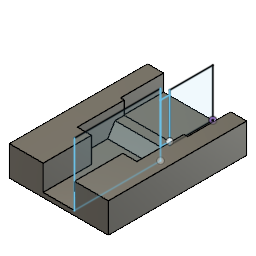
Universal Power v1 (Autodesk Fusion 360 design; units mm, degrees)
Autodesk Fusion 360 part; units mm, degrees
sketch "Sketch1" plane through (0, 0, 0) normal (1, 0, 0) x (0, 0, -1)
  line L0 (0, 0) -> (-18.75, 0)
  line L1 (-18.75, 0) -> (-18.75, 20.75)
  line L2 (-18.75, 20.75) -> (0, 20.75)
  line L3 (0, 20.75) -> (0, 0)
  line L4 (-18.75, 20.75) -> (-18.75, 19)
  line L5 (-18.75, 0) -> (-18.75, 1.4)
  line L6 (-18.75, 19) -> (-22.75, 19)
  line L7 (-22.75, 19) -> (-22.75, 1.4)
  line L8 (-22.75, 1.4) -> (-18.75, 1.4)
  line L9 (-18.75, 1.4) -> (-18.75, 19)
  line L10 (-22.75, 19) -> (-22.75, 23.35)
  line L11 (-22.75, 1.4) -> (-22.75, -3.85)
  line L12 (-22.75, 23.35) -> (-60.15, 23.35)
  line L13 (-60.15, 23.35) -> (-60.15, -3.85)
  line L14 (-60.15, -3.85) -> (-22.75, -3.85)
  line L15 (-22.75, -3.85) -> (-22.75, 23.35)
  dimension "d1" = 18.75
  dimension "d2" = 20.75
  dimension "d4" = 1.75
  dimension "d6" = 4
  dimension "d7" = 4.35
  dimension "d9" = 37.4
  constraint horizontal L0
  constraint vertical L1
  constraint horizontal L2
  constraint vertical L3
  constraint coincident L0.start L3.end
  constraint horizontal L6
  constraint vertical L7
  constraint horizontal L8
  constraint vertical L9
  constraint horizontal L12
  constraint vertical L13
  constraint horizontal L14
  constraint vertical L15
  measures "d1" distance of L0.start L0.end
  measures "d2" distance of L0.start L2.end
  measures "d4" distance of L1.end L4.end
  measures "d6" distance of L4.end L6.end
  measures "d7" distance of L6.end L10.end
  measures "d9" distance of L10.end L12.end
sketch "Sketch3" plane through (0, 0, 0) normal (1, 0, 0) x (0, 0, -1)
  line L0 (-60.15, -3.85) -> (-60.15, 7.15)
  line L1 (-60.15, 7.15) -> (-39.15, 7.15)
  line L2 (-60.15, -3.85) -> (-22.75, -3.85)
  line L3 (-39.15, 7.15) -> (-39.15, -3.85)
  point P0 (-60.15, -3.85)
  dimension "d10" = 11
  dimension "d11" = 21
  constraint coincident P0 L0.start
  constraint coincident L2 L3.end
  constraint perpendicular L1 L3
  measures "d10" distance of P0 L0.end
  measures "d11" distance of L0.end L1.end
extrude "Extrude1" add sketch "Sketch3" along normal blind 6.15 makes body 1
sketch "Sketch4" plane through (6.15, 0, 0) normal (1, 0, 0) x (0, 0, -1)
  line L0 (-60.15, -3.85) -> (-39.15, -3.85)
  line L1 (-39.15, -3.85) -> (-39.15, 7.15)
  line L2 (-39.15, 7.15) -> (-60.15, 7.15)
  line L3 (-60.15, 7.15) -> (-60.15, -3.85)
  line L4 (-60.15, -3.85) -> (-18.75, -3.85)
  line L5 (-18.75, -3.85) -> (-18.75, 7.15)
  line L6 (-18.75, 7.15) -> (-60.15, 7.15)
  line L7 (-60.15, 7.15) -> (-60.15, -3.85)
  line L8 (-18.75, 1.4) -> (-18.75, 19)
  constraint horizontal L4
  constraint vertical L5
  constraint horizontal L6
  constraint vertical L7
  constraint coincident L5.end L8
  constraint coincident L0.start L3.end
extrude "Extrude2" add sketch "Sketch4" along normal blind 1.6 bodies 1
sketch "Sketch5" plane through (7.75, 0, 0) normal (1, 0, 0) x (0, 0, -1)
  line L0 (-18.75, -3.85) -> (-18.75, 7.15)
  line L1 (-18.75, 7.15) -> (-60.15, 7.15)
  line L2 (-60.15, 7.15) -> (-60.15, -3.85)
  line L3 (-60.15, -3.85) -> (-18.75, -3.85)
  line L4 (-60.15, -3.85) -> (0, -3.85)
  line L5 (0, -3.85) -> (0, 7.15)
  line L6 (0, 7.15) -> (-60.15, 7.15)
  line L7 (-60.15, 7.15) -> (-60.15, -3.85)
  line L8 (0, 20.75) -> (0, 0)
  constraint horizontal L4
  constraint vertical L5
  constraint horizontal L6
  constraint vertical L7
  constraint coincident L5.end L8
  constraint coincident L2.end L3.start
extrude "Extrude3" add sketch "Sketch5" along normal blind 7 bodies 1
sketch "Sketch6" plane through (0, 0, 60.15) normal (0, 0, 1) x (1, 0, 0)
  line L0 (0, 7.15) -> (0, -3.85)
  line L1 (0, -3.85) -> (14.75, -3.85)
  line L2 (14.75, -3.85) -> (14.75, 7.15)
  line L3 (14.75, 7.15) -> (0, 7.15)
  line L4 (0, -3.85) -> (-13.6, -3.85)
  dimension "d18" = 13.6
  constraint coincident L0.end L1.start
  measures "d18" distance of L0.end L4.end
extrude "Extrude4" add sketch "Sketch3" along normal blind -14 and the other way blind 13.6 separate body makes body 2
extrude "Extrude5" add 1 faces at (-14, -0.1833, 46.15) along direction (-1, 0, 0) blind 6.15 on bodies 2 bodies 2
extrude "Extrude6" cut 1 faces at (-20.15, -0.1833, 46.15) along direction (1, 0, 0) blind 0.4 on bodies 2 bodies 2
sketch "Sketch7" plane through (-19.75, 0, 0) normal (-1, 0, 0) x (0, 0, 1)
  line L0 (39.15, -3.85) -> (60.15, -3.85)
  line L1 (60.15, -3.85) -> (60.15, 7.15)
  line L2 (60.15, 7.15) -> (39.15, 7.15)
  line L3 (39.15, 7.15) -> (39.15, -3.85)
  line L4 (60.15, 7.15) -> (18.75, 7.15)
  line L5 (18.75, 7.15) -> (18.75, -3.85)
  line L6 (18.75, -3.85) -> (60.15, -3.85)
  line L7 (60.15, -3.85) -> (60.15, 7.15)
  point P0 (18.75, -3.85)
  constraint horizontal L4
  constraint vertical L5
  constraint horizontal L6
  constraint vertical L7
  constraint coincident P0 L5.end
  constraint coincident L1.end L2.start
extrude "Extrude7" add sketch "Sketch7" along normal blind 1.6 bodies 2
sketch "Sketch8" plane through (-21.35, 0, 0) normal (-1, 0, 0) x (0, 0, 1)
  line L0 (60.15, -3.85) -> (60.15, 7.15)
  line L1 (60.15, 7.15) -> (18.75, 7.15)
  line L2 (18.75, 7.15) -> (18.75, -3.85)
  line L3 (18.75, -3.85) -> (60.15, -3.85)
  line L4 (60.15, 7.15) -> (0, 7.15)
  line L5 (0, 7.15) -> (0, -3.85)
  line L6 (0, -3.85) -> (60.15, -3.85)
  line L7 (60.15, -3.85) -> (60.15, 7.15)
  point P0 (0, -3.85)
  constraint horizontal L4
  constraint vertical L5
  constraint horizontal L6
  constraint vertical L7
  constraint coincident P0 L5.end
  constraint coincident L0.end L1.start
extrude "Extrude8" add sketch "Sketch8" along normal blind 7 bodies 2
sketch "Sketch9" plane through (0, 0, 0) normal (1, 0, 0) x (0, 0, -1)
  line L0 (-60.15, -3.85) -> (-25.95, -3.85)
  line L1 (-25.95, -3.85) -> (-22.75, 1.4)
  line L2 (-22.75, 1.4) -> (-18.75, 1.4)
  line L3 (-18.75, 1.4) -> (-18.75, 0)
  line L4 (-18.75, 0) -> (0, 0)
  line L5 (-25.95, -3.85) -> (0, -3.85)
  line L6 (0, -3.85) -> (0, 0)
  point P0 (-60.15, -3.85)
  point P1 (-22.75, 1.4)
  point P2 (-18.75, 1.4)
  point P3 (-18.75, 0)
  dimension "d31" = 34.2
  constraint coincident P0 L0.start
  constraint coincident P1 L1.end
  constraint coincident P2 L2.end
  constraint parallel L0 L2
  constraint coincident P3 L3.end
  constraint coincident L4.end L6.end
  constraint parallel L0 L5
  constraint perpendicular L4 L6
  measures "d31" distance of P0 L0.end
extrude "Extrude9" add sketch "Sketch9" along normal blind 8 and the other way blind 24 bodies 1 2
sketch "Sketch10" plane through (0, -3.85, 0) normal (0, -1, 0) x (1, 0, 0)
  line L0 (-19.75, 25.95) -> (-19.75, 39.15)
  line L1 (-19.75, 39.15) -> (-13.6, 39.15)
  line L2 (-13.6, 39.15) -> (-13.6, 60.15)
  line L3 (-13.6, 60.15) -> (-28.35, 60.15)
  line L4 (-28.35, 60.15) -> (-28.35, 0)
  line L5 (-28.35, 0) -> (14.75, 0)
  line L6 (14.75, 0) -> (14.75, 60.15)
  line L7 (14.75, 60.15) -> (0, 60.15)
  line L8 (0, 60.15) -> (0, 39.15)
  line L9 (0, 39.15) -> (6.15, 39.15)
  line L10 (6.15, 39.15) -> (6.15, 25.95)
  line L11 (6.15, 25.95) -> (-19.75, 25.95)
  line L12 (-28.35, 60.15) -> (14.75, 60.15)
  line L13 (14.75, 60.15) -> (14.75, 0)
  line L14 (14.75, 0) -> (-28.35, 0)
  line L15 (-28.35, 0) -> (-28.35, 60.15)
  constraint horizontal L12
  constraint vertical L13
  constraint horizontal L14
  constraint vertical L15
  constraint coincident L5.end L6.start
  constraint coincident L3.end L4.start
extrude "Extrude10" add sketch "Sketch10" along normal blind 2 bodies 1
